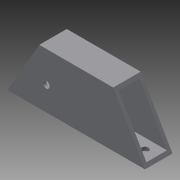
# Autodesk Inventor part: MotorSupport
Saved by Autodesk Inventor 2013 (Build 170138000, 138)
## iProperties
Created: 2014-01-22
Part Number: MotorSupport
Material: Generic
Document SubType Name: Modeling
Designer: 215152
Density: 1 g/cm^3
Author: 215152
Autodesk Inventor part; units mm, degrees
ref_plane "YZ Plane" through (0, 0, 0) normal (1, 0, 0) x (0, 1, 0)
ref_plane "XZ Plane" through (0, 0, 0) normal (0, 1, 0) x (-1, 0, 0)
ref_plane "XY Plane" through (0, 0, 0) normal (0, 0, 1) x (1, 0, 0)
sketch "Sketch1" plane through (0, 0, 0) normal (0, 0, 1) x (1, 0, 0)
  line L0 (0, 0) -> (127, 0)
  line L1 (127, 0) -> (127, 50.8)
  line L2 (127, 50.8) -> (0, 50.8)
  line L3 (0, 50.8) -> (0, 0)
  dimension "d0" = 127
  dimension "d1" = 50.8
  constraints: 8 end point, 2 parallel, 1 horizontal, 1 perpendicular
  measures "d0" distance of L2.end L1.end
  measures "d1" distance of L1.end L0.end
extrude "Extrusion1" add sketch "Sketch1" along normal blind 25.4
sketch "Sketch2" plane through (127, 0, 0) normal (1, 0, 0) x (0, 0, -1)
  line L0 (-22.225, 3.175) -> (-3.175, 3.175)
  line L1 (-3.175, 3.175) -> (-3.175, 47.625)
  line L2 (-3.175, 47.625) -> (-22.225, 47.625)
  line L3 (-22.225, 47.625) -> (-22.225, 3.175)
  dimension "d4" = 19.05
  dimension "d5" = 44.45
  constraints: 8 end point, 2 parallel, 1 horizontal, 1 perpendicular
  measures "d4" distance of L2.end L1.end
  measures "d5" distance of L1.end L0.end
extrude "Extrusion2" cut sketch "Sketch2" against normal blind 2514.6
sketch "Sketch3" plane through (0, 0, 25.4) normal (0, 0, 1) x (1, 0, 0)
  line L0 (127, 0) -> (127, 50.8) projected
  line L1 (127, 50.8) -> (0, 50.8) projected
  line L2 (0, 50.8) -> (0, 0) projected
  line L3 (0, 0) -> (29.3294, 50.8)
  line L4 (0, 0) -> (58.6588, 0) construction
  line L5 (127, 0) -> (97.6706, 50.8)
  line L6 (127, 0) -> (185.6588, 0) construction
  dimension "d8" = 60
  dimension "d9" = 120
  constraints: 8 end point, 2 equal length, 2 horizontal, 2 point on line
  measures "d8" angle of L4 L3
  measures "d9" angle of L6 L5
extrude "Extrusion3" cut sketch "Sketch3" against normal blind 2514.6
sketch "Sketch4" plane through (0, 0, 0) normal (0, -1, 0) x (1, 0, 0)
  circle A0 centre (12.7, 12.7) radius 3.175
  circle A1 centre (114.3, 12.7) radius 3.175
  dimension "d12" = 6.35
  dimension "d13" = 6.35
  constraints: 2 centre point
  measures "d12" diameter of A0
  measures "d13" diameter of A1
extrude "Extrusion4" cut sketch "Sketch4" against normal blind 2514.6
sketch "Sketch5" plane through (0, 0, 25.4) normal (0, 0, 1) x (1, 0, 0)
  line L0 (0, 0) -> (127, 0) projected
  line L1 (29.3294, 50.8) -> (97.6706, 50.8)
  line L2 (97.6706, 50.8) -> (97.6706, 0)
  line L3 (97.6706, 0) -> (29.3294, 0)
  line L4 (29.3294, 0) -> (29.3294, 50.8)
  line L5 (29.3294, 0) -> (35.6794, 0)
  line L6 (35.6794, 0) -> (35.6794, 22.2377)
  line L7 (35.6794, 22.2377) -> (97.6706, 22.2377)
  line L8 (97.6706, 22.2377) -> (84.9706, 22.2377)
  circle A0 centre (35.6794, 22.2377) radius 3.175
  dimension "d16" = 6.35
  dimension "d17" = 22.2377
  dimension "d18" = 90
  dimension "d19" = 12.7
  dimension "d20" = 6.35
  constraints: 16 end point, 4 point on line, 3 perpendicular, 2 parallel, 1 centre point, 1 coincident, 1 horizontal
  measures "d16" distance of L3.end L5.end
  measures "d17" distance of L5.end L6.end
  measures "d18" angle of L6 L5
  measures "d19" distance of L7.end L8.end
  measures "d20" diameter of A0
extrude "Extrusion5" cut sketch "Sketch5" against normal blind 2514.6 contours A0 L7 L6 | L6 L7 A0
body "Solid1"
